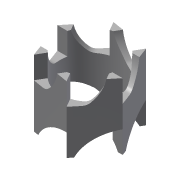
# Autodesk Inventor part: SPRING NUT1
Saved by Autodesk Inventor 2014 (Build 180170000, 170)
## iProperties
Created: 2014-12-19
Part Number: SPRING NUT1
Material: Steel, Mild
Document SubType Name: Modeling
Designer: Ebrahim
Density: 7.86 g/cm^3
Appearance: Steel
Mass: 4.5993 g
Surface Area: 11.347 cm^2
Volume: 0.585152 cm^3
Author: Ebrahim
Autodesk Inventor part; units mm, degrees
sketch "Sketch1" plane through (0, 0, 0) normal (1, 0, 0) x (0, 1, 0)
  circle A0 centre (0, 0) radius 9
  dimension "d31" = 18
  constraints: 2 coincident, 1 centre point, 1 other
  measures "d31" diameter of A0
extrude "Extrusion1" add sketch "Sketch1" against normal blind 15
hole "Hole1" at (0, 0, 0) direction (-1, 0, 0) diameter 13.5 end through all
ref_plane "Work Plane1" through (0, 0, 1.5) normal (0, 0, 1) x (1, 0, 0)
ref_plane "Work Plane2" through (-5, -9, 1.5) normal (0, -1, 0) x (1, 0, 0)
sketch "Sketch4" plane through (-5, -9, 1.5) normal (0, -1, 0) x (1, 0, 0)
  line L0 (-10, -3) -> (-5, -3)
  line L1 (-10, 0) -> (-10, -6) construction
  line L2 (-40.0446, 0) -> (21.4016, 0) construction
  line L3 (-5, 0) -> (-5, 0.1987) construction
  arc A0 (-10, -6) -> (-5.0454, -0.225) centre (-12.8638, 1.4698) ccw construction
  arc A1 (-5.0454, -0.225) -> (-5, 0.1987) centre (-7, 0.1987) ccw construction
  line L4 (-10, -3) -> (-10, 3)
  line L5 (-5, -3) -> (-5, -0.7378)
  arc A2 (-5.5557, 0.6457) -> (-10, 3) centre (-11.3329, -4.8882) ccw
  arc A3 (-5, -0.7378) -> (-5.5557, 0.6457) centre (-7, -0.7378) ccw
  line L6 (-10, -8.25) -> (-10, 5.25) construction
  line L7 (-10, -8.25) -> (-10, 5.25) construction
  line L8 (-10, 7.5) -> (-10, -10.5) construction
  line L9 (-10, 7.5) -> (12.6236, 7.5)
  line L10 (-5, -1.5) -> (12.6236, -1.5)
  line L11 (-10, 7.5) -> (5, 7.5)
  line L12 (-2.5, 7.5) -> (-2.5, -13.092)
  line L13 (35.0446, 0) -> (-26.4016, 0) construction
  arc A4 (0.0454, -0.225) -> (5, -6) centre (7.8638, 1.4698) ccw construction
  arc A5 (0.0099, 0) -> (0.0454, -0.225) centre (2, 0.1987) ccw
  line L14 (5, 0.1987) -> (5, -10.5) construction
  line L15 (5, -6) -> (5, 0) construction
  line L16 (0.0099, 0) -> (5, 0) construction
  line L17 (-10, 3) -> (6.7233, 3)
  arc A6 (0.0099, -3) -> (0.0454, -3.225) centre (2, -2.8013) ccw
  arc A7 (0.0454, -3.225) -> (5, -9) centre (7.8638, -1.5302) ccw
  line L18 (5, -9) -> (5, -3)
  line L19 (0.0099, -3) -> (5, -3)
  line L20 (-10, -3) -> (-5, -3)
  line L21 (0.0099, -3) -> (12.6236, -3)
  point P0 (5, -1.5)
  point P1 (-4.9623, 0.2185)
  point P2 (-5, 0)
  point P3 (-4.9623, -0.2185)
  point P4 (-5, 0)
  point P5 (-0.0377, 0.2185)
  point P6 (0, 0)
  point P7 (-0.0377, -0.2185)
  point P8 (0, 0)
  point P9 (5, 0)
  dimension "d43" = 6
  dimension "d47" = 2
  dimension "d49" = 8
  dimension "d76" = 18
  dimension "d77" = 9
  dimension "d78" = 6
  dimension "d79" = 8
  dimension "d80" = 2
  dimension "d81" = 5
  dimension "d82" = 1.5
  dimension "d84" = 15
  constraints: 36 end point, 21 point on circle, 14 symmetric about line, 8 centre point, 5 point on line, 4 parallel, 3 perpendicular, 2 tangent, 1 midpoint, 2 other
  measures "d43" distance of L1.start L1.end
  measures "d47" radius of A1
  measures "d49" radius of A0
  measures "d76" distance of L8.start L8.end
  measures "d77" distance between parallel lines of L10 L9
  measures "d78" distance of L0.start L4.end
  measures "d79" radius of A2
  measures "d80" radius of A3
  measures "d81" distance between parallel lines of L5 L4
  measures "d82" distance between parallel lines of L0 L10
  measures "d84" distance of L8.start L11.end
extrude "Extrusion7" cut sketch "Sketch4" against normal blind 10 contours L4 A2 A3 L5 L0 | L19 L18 A7 A6
pattern_circular "Circular Pattern3" count 6 over 360 about axis through (-10, 0, 0) along (1, 0, 0) of "Extrusion7"
ref_plane "Work Plane3" through (-7.5, 0, 0) normal (1, 0, 0) x (0, 0, -1)
sketch "Sketch6" plane through (-15, 0, 0) normal (-1, 0, 0) x (0, 0, 1)
  line L0 (-6.9352, 5.7361) -> (1.5, 8.8741)
  line L1 (6.9352, -5.7361) -> (4.9495, -4.5896) construction
  line L2 (4.5, -5.0312) -> (4.5, -7.7942) construction
  arc A0 (4.5, -7.7942) -> (6.9352, -5.7361) centre (0, 0) ccw construction
  line L3 (8.4352, 3.138) -> (6.4495, 1.9916) construction
  line L4 (6.6071, 1.3815) -> (9, 0) construction
  arc A1 (9, 0) -> (8.4352, 3.138) centre (0, 0) ccw construction
  line L5 (2.1071, 6.4127) -> (4.5, 7.7942) construction
  arc A2 (4.5, 7.7942) -> (1.5, 8.8741) centre (0, 0) ccw construction
  line L6 (1.5, 8.8741) -> (1.5, 6.5812) construction
  line L7 (-4.5, 5.0312) -> (-4.5, 7.7942) construction
  arc A3 (-4.5, 7.7942) -> (-6.9352, 5.7361) centre (0, 0) ccw construction
  line L8 (-6.9352, 5.7361) -> (-4.9495, 4.5896) construction
  line L9 (-6.6071, -1.3815) -> (-9, 0) construction
  arc A4 (-9, 0) -> (-8.4352, -3.138) centre (0, 0) ccw construction
  line L10 (-8.4352, -3.138) -> (-6.4495, -1.9916) construction
  line L11 (-2.1071, -6.4127) -> (-4.5, -7.7942) construction
  arc A5 (-4.5, -7.7942) -> (-1.5, -8.8741) centre (0, 0) ccw construction
  line L12 (-1.5, -8.8741) -> (-1.5, -6.5812) construction
  line L13 (0, 0) -> (-6.9352, 5.7361)
  line L14 (1.5, 8.8741) -> (0, 0)
  circle A6 centre (0, 0) radius 9
  line L15 (-8.4352, -3.138) -> (-6.9352, 5.7361)
  line L16 (0, 0) -> (-8.4352, -3.138)
  line L17 (-6.9352, 5.7361) -> (0, 0)
  line L18 (-1.5, -8.8741) -> (-8.4352, -3.138)
  line L19 (0, 0) -> (-1.5, -8.8741)
  line L20 (-8.4352, -3.138) -> (0, 0)
  line L21 (6.9352, -5.7361) -> (-1.5, -8.8741)
  line L22 (0, 0) -> (6.9352, -5.7361)
  line L23 (-1.5, -8.8741) -> (0, 0)
  line L24 (8.4352, 3.138) -> (6.9352, -5.7361)
  line L25 (0, 0) -> (8.4352, 3.138)
  line L26 (6.9352, -5.7361) -> (0, 0)
  line L27 (1.5, 8.8741) -> (8.4352, 3.138)
  line L28 (0, 0) -> (1.5, 8.8741)
  line L29 (8.4352, 3.138) -> (0, 0)
  arc A7 (-2.1071, -6.4127) -> (-1.5, -6.5812) centre (0, 0) ccw projected
  arc A8 (-6.6071, -1.3815) -> (-6.4495, -1.9916) centre (0, 0) ccw projected
  arc A9 (-4.5, 5.0312) -> (-4.9495, 4.5896) centre (0, 0) ccw projected
  arc A10 (2.1071, 6.4127) -> (1.5, 6.5812) centre (0, 0) ccw projected
  arc A11 (6.6071, 1.3815) -> (6.4495, 1.9916) centre (0, 0) ccw projected
  arc A12 (4.5, -5.0312) -> (4.9495, -4.5896) centre (0, 0) ccw projected
  dimension "d72" = 360
  constraints: 36 end point, 8 point on line, 2 coincident, 1 point on circle, 46 other
extrude "Extrusion11" cut sketch "Sketch6" against normal through all contours A6 L0 | L15 A6 | A6 L27 | L18 A6 | A6 L24 | L21 A6
body "Solid1"
